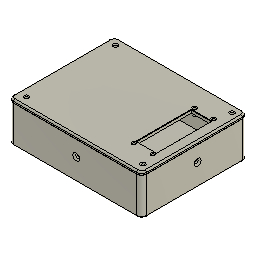
3d_case (Autodesk Fusion 360 design; units mm, degrees)
Autodesk Fusion 360 part; units mm, degrees
note: some values were not read from the file. Chosen so that the rebuilt part matches the saved one: which bodies a step acts on.
sketch "Sketch1" plane through (0, 0, 0) normal (0, 0, 1) x (1, 0, 0)
  line L0 (25.4, 25.4) -> (171.785, 25.4)
  line L1 (171.785, 25.4) -> (171.785, 136.054)
  line L2 (171.785, 136.054) -> (25.4, 136.054)
  line L3 (25.4, 136.054) -> (25.4, 25.4)
  line L4 (17.9, 15.4) -> (179.285, 15.4)
  line L5 (181.785, 17.9) -> (181.785, 143.554)
  line L6 (179.285, 146.054) -> (17.9, 146.054)
  line L7 (15.4, 143.554) -> (15.4, 17.9)
  arc A0 (17.9, 146.054) -> (15.4, 143.554) centre (17.9, 143.554) ccw
  arc A1 (15.4, 17.9) -> (17.9, 15.4) centre (17.9, 17.9) ccw
  arc A2 (179.285, 15.4) -> (181.785, 17.9) centre (179.285, 17.9) ccw
  arc A3 (181.785, 143.554) -> (179.285, 146.054) centre (179.285, 143.554) ccw
  line L8 (11.4, 143.554) -> (11.4, 17.9)
  arc A4 (11.4, 17.9) -> (17.9, 11.4) centre (17.9, 17.9) ccw
  line L9 (17.9, 11.4) -> (179.285, 11.4)
  arc A5 (179.285, 11.4) -> (185.785, 17.9) centre (179.285, 17.9) ccw
  line L10 (185.785, 17.9) -> (185.785, 143.554)
  arc A6 (185.785, 143.554) -> (179.285, 150.054) centre (179.285, 143.554) ccw
  line L11 (179.285, 150.054) -> (17.9, 150.054)
  arc A7 (17.9, 150.054) -> (11.4, 143.554) centre (17.9, 143.554) ccw
  dimension "d2" = 2.5
  dimension "d3" = 4
  constraint parallel L0 L4
  constraint parallel L1 L5
  constraint parallel L2 L6
  constraint parallel L3 L7
  constraint tangent L6 A0
  constraint tangent L7 A0
  constraint tangent L4 A1
  constraint tangent L7 A1
  constraint equal A0 A1
  constraint tangent L4 A2
  constraint tangent L5 A2
  constraint equal A0 A2
  constraint tangent L5 A3
  constraint tangent L6 A3
  constraint equal A0 A3
  measures "d2" radius of A0
extrude "Extrude1" add sketch "Sketch1" along normal blind 5 and the other way blind 40 contours L8 A4 L9 A5 L10 A6 L11 A7 makes body 1
extrude "Extrude2" add sketch "Sketch1" against normal blind 4 from surface at -40 contours L0 L1 L2 L3 | L4 L5 L6 L7 A0 A1 A2 A3 | L8 A4 L9 A5 L10 A6 L11 A7 bodies 1
extrude "Extrude3" add sketch "Sketch1" along normal blind 4 from surface at 5 separate body contours L0 L1 L2 L3 | L4 L5 L6 L7 A0 A1 A2 A3 | L8 A4 L9 A5 L10 A6 L11 A7 makes body 2
fillet "Fillet1" radius 2 16 edges at (98.5925, 150.054, -44) (183.8812, 148.1502, -44) (185.785, 80.727, -44) (183.8812, 13.3038, -44) (98.5925, 11.4, -44) (13.3038, 13.3038, -44) (11.4, 80.727, -44) (13.3038, 148.1502, -44) (11.4, 80.727, 9) (13.3038, 13.3038, 9) (98.5925, 11.4, 9) (183.8812, 13.3038, 9) (185.785, 80.727, 9) (183.8812, 148.1502, 9) (98.5925, 150.054, 9) (13.3038, 148.1502, 9) on bodies 1 2
fillet "Fillet2" radius 0.25 8 edges at (185.785, 80.727, 5) (183.8812, 148.1502, 5) (98.5925, 150.054, 5) (13.3038, 148.1502, 5) (11.4, 80.727, 5) (13.3038, 13.3038, 5) (98.5925, 11.4, 5) (183.8812, 13.3038, 5) on bodies 2
sketch "Sketch2" plane through (0, 0, 5) normal (0, 0, 1) x (-1, 0, 0)
  arc A0 (-181.785, -143.554) -> (-179.285, -146.054) centre (-179.285, -143.554) ccw
  line L0 (-181.785, -143.554) -> (-181.785, -17.9)
  arc A1 (-179.285, -15.4) -> (-181.785, -17.9) centre (-179.285, -17.9) ccw
  line L1 (-179.285, -15.4) -> (-17.9, -15.4)
  arc A2 (-15.4, -17.9) -> (-17.9, -15.4) centre (-17.9, -17.9) ccw
  line L2 (-15.4, -17.9) -> (-15.4, -143.554)
  arc A3 (-17.9, -146.054) -> (-15.4, -143.554) centre (-17.9, -143.554) ccw
  line L3 (-17.9, -146.054) -> (-179.285, -146.054)
  arc A4 (-17.9, -150.054) -> (-11.4, -143.554) centre (-17.9, -143.554) ccw
  line L4 (-11.4, -143.554) -> (-11.4, -17.9)
  arc A5 (-11.4, -17.9) -> (-17.9, -11.4) centre (-17.9, -17.9) ccw
  line L5 (-17.9, -11.4) -> (-179.285, -11.4)
  arc A6 (-179.285, -11.4) -> (-185.785, -17.9) centre (-179.285, -17.9) ccw
  line L6 (-185.785, -17.9) -> (-185.785, -143.554)
  arc A7 (-185.785, -143.554) -> (-179.285, -150.054) centre (-179.285, -143.554) ccw
  line L7 (-179.285, -150.054) -> (-17.9, -150.054)
  arc A8 (-17.9, -148.054) -> (-13.4, -143.554) centre (-17.9, -143.554) ccw
  line L8 (-13.4, -17.9) -> (-13.4, -143.554)
  arc A9 (-13.4, -17.9) -> (-17.9, -13.4) centre (-17.9, -17.9) ccw
  line L9 (-179.285, -13.4) -> (-17.9, -13.4)
  arc A10 (-179.285, -13.4) -> (-183.785, -17.9) centre (-179.285, -17.9) ccw
  line L10 (-183.785, -143.554) -> (-183.785, -17.9)
  arc A11 (-183.785, -143.554) -> (-179.285, -148.054) centre (-179.285, -143.554) ccw
  line L11 (-17.9, -148.054) -> (-179.285, -148.054)
  dimension "d18" = -2
extrude "Extrude4" cut sketch "Sketch2" against normal blind 2 contours A8 L8 A9 L9 A10 L10 A11 L11 bodies 1
extrude "Extrude5" add sketch "Sketch2" against normal blind 2 contours A8 L8 A9 L9 A10 L10 A11 L11 bodies 2
fillet "Fillet3" radius 0.2 8 edges at (98.5925, 148.054, 3) (182.467, 146.736, 3) (183.785, 80.727, 3) (182.467, 14.718, 3) (98.5925, 13.4, 3) (14.718, 14.718, 3) (13.4, 80.727, 3) (14.718, 146.736, 3) on bodies 2
sketch "Sketch10" plane through (0, 0, 9) normal (0, 0, 1) x (-1, 0, 0)
  line L0 (-13.4, -143.554) -> (-13.4, -17.9)
  arc A0 (-13.4, -17.9) -> (-17.9, -13.4) centre (-17.9, -17.9) ccw
  line L1 (-17.9, -13.4) -> (-179.285, -13.4)
  arc A1 (-179.285, -13.4) -> (-183.785, -17.9) centre (-179.285, -17.9) ccw
  line L2 (-183.785, -17.9) -> (-183.785, -143.554)
  arc A2 (-183.785, -143.554) -> (-179.285, -148.054) centre (-179.285, -143.554) ccw
  line L3 (-179.285, -148.054) -> (-17.9, -148.054)
  arc A3 (-17.9, -148.054) -> (-13.4, -143.554) centre (-17.9, -143.554) ccw
  line L4 (-158.9282, -148.054) -> (-158.9282, -13.4) construction
  line L5 (-172.0282, -44.727) -> (-145.8282, -44.727)
  line L6 (-145.8282, -44.727) -> (-145.8282, -116.727)
  line L7 (-145.8282, -116.727) -> (-172.0282, -116.727)
  line L8 (-172.0282, -116.727) -> (-172.0282, -44.727)
  line L9 (-172.0282, -44.727) -> (-145.8282, -116.727) construction
  line L10 (-145.8282, -44.727) -> (-172.0282, -116.727) construction
  point P0 (-158.9282, -80.727)
  dimension "d87" = 26.2
  dimension "d88" = 72
  constraint coincident L3 L4.start
  constraint coincident L1 L4.end
  constraint perpendicular L1 L4
  constraint horizontal L5
  constraint perpendicular L5 L6
  constraint parallel L5 L7
  constraint parallel L6 L8
  constraint coincident L9 P0
  constraint coincident L10 P0
  constraint midpoint L4 P0
  measures "d87" distance of L6.end L7.end
  measures "d88" distance of L5.end L6.end
sketch "Sketch4" plane through (11.4, 0, 0) normal (-1, 0, 0) x (0, -1, 0)
  line L0 (-143.554, -42) -> (-17.9, -42)
  line L1 (-17.9, -42) -> (-17.9, 5)
  line L2 (-17.9, 5) -> (-143.554, 5)
  line L3 (-143.554, 5) -> (-143.554, -42)
  line L4 (-143.554, -18.5) -> (-17.9, -18.5) construction
  line L5 (-66.727, -27) -> (-94.727, -27)
  line L6 (-94.727, -27) -> (-94.727, -10)
  line L7 (-94.727, -10) -> (-66.727, -10)
  line L8 (-66.727, -10) -> (-66.727, -27)
  line L9 (-66.727, -27) -> (-94.727, -10) construction
  line L10 (-94.727, -27) -> (-66.727, -10) construction
  circle A0 centre (-80.5064, -7.1438) radius 1
  circle A1 centre (-81, -30) radius 1
  point P0 (-80.727, -18.5)
  dimension "d29" = 28
  dimension "d30" = 17
  dimension "d31" = 2
  dimension "d32" = 2
  constraint midpoint L3 L4.start
  constraint midpoint L1 L4.end
  constraint horizontal L5
  constraint perpendicular L5 L6
  constraint parallel L5 L7
  constraint parallel L6 L8
  constraint coincident L9 P0
  constraint coincident L10 P0
  constraint midpoint L4 P0
  measures "d29" distance of L6.end L7.end
  measures "d30" distance of L5.end L6.end
  measures "d31" diameter of A0
  measures "d32" diameter of A1
extrude "Extrude12" cut sketch "Sketch10" against normal blind 10 contours L5 L6 L7 L8 bodies 2
extrude "Extrude7" cut sketch "Sketch4" against normal blind 14 contours L5 L6 L7 L8 | A0 | A1 bodies 1
sketch "Sketch5" plane through (181.785, 0, 0) normal (-1, 0, 0) x (0, -1, 0)
  line L0 (-17.9, 3) -> (-143.554, 3)
  line L1 (-143.554, 3) -> (-143.554, -40)
  line L2 (-143.554, -40) -> (-17.9, -40)
  line L3 (-17.9, -40) -> (-17.9, 3)
  circle A0 centre (-118.7918, -5.4) radius 1
  circle A1 centre (-41.7918, -5.4) radius 1
  circle A2 centre (-118.7918, -31.4) radius 1
  circle A3 centre (-41.7918, -31.4) radius 1
  circle A4 centre (-118.7918, -5.4) radius 1.75
  circle A5 centre (-41.7918, -5.4) radius 1.75
  circle A6 centre (-118.7918, -31.4) radius 1.75
  circle A7 centre (-41.7918, -31.4) radius 1.75
  dimension "d35" = 2
  dimension "d38" = 77
  dimension "d39" = -26
  dimension "d40" = 3.5
  constraint concentric A0 A4
  measures "d35" diameter of A0
  measures "d40" diameter of A4
sketch "Sketch6" plane through (0, 0, 0) normal (0, 0, 1) x (-1, 0, 0)
  line L0 (-25.4, -25.4) -> (-171.785, -25.4)
  line L1 (-171.785, -25.4) -> (-171.785, -136.054)
  line L2 (-171.785, -136.054) -> (-25.4, -136.054)
  line L3 (-25.4, -136.054) -> (-25.4, -25.4)
  circle A0 centre (-32, -130) radius 1.25
  circle A1 centre (-32, -130) radius 2
  circle A2 centre (-165, -130) radius 1.25
  circle A3 centre (-165, -130) radius 2
  circle A4 centre (-32, -33) radius 1.25
  circle A5 centre (-32, -33) radius 2
  circle A6 centre (-165, -33) radius 1.25
  circle A7 centre (-165, -33) radius 2
  dimension "d43" = 2.5
  dimension "d46" = -133
  dimension "d47" = 97
  constraint concentric A0 A1
  measures "d43" diameter of A0
extrude "Extrude9" add sketch "Sketch6" against normal up to surface (39.59 mm away) from surface at -0.41 separate body contours A1 | A3 | A5 | A7 makes body 3 at (163.0025, 129.9003, -13.6067) makes body 4 at (164.1774, 31.177, -26.8033) makes body 5 at (33.3965, 31.5683, -26.8033) makes body 6 at (30.8325, 128.3761, -26.8033)
combine "Combine1" operation add target body 1 tool bodies 3 4 5 6
sketch "Sketch7" plane through (0, 0, -40) normal (0, 0, 1) x (-1, 0, 0)
  circle A0 centre (-32, -33) radius 2
  circle A1 centre (-165, -130) radius 2
  line L0 (-179.285, -146.054) -> (-17.9, -146.054)
  arc A2 (-17.9, -146.054) -> (-15.4, -143.554) centre (-17.9, -143.554) ccw
  line L1 (-15.4, -143.554) -> (-15.4, -17.9)
  arc A3 (-15.4, -17.9) -> (-17.9, -15.4) centre (-17.9, -17.9) ccw
  line L2 (-17.9, -15.4) -> (-179.285, -15.4)
  arc A4 (-179.285, -15.4) -> (-181.785, -17.9) centre (-179.285, -17.9) ccw
  line L3 (-181.785, -17.9) -> (-181.785, -143.554)
  arc A5 (-181.785, -143.554) -> (-179.285, -146.054) centre (-179.285, -143.554) ccw
  circle A6 centre (-165, -33) radius 2
  circle A7 centre (-32, -130) radius 2
  circle A8 centre (-23, -140) radius 1.25
  circle A9 centre (-23, -140) radius 2
  circle A10 centre (-176, -140) radius 2
  circle A11 centre (-176, -140) radius 1.25
  circle A12 centre (-23, -23) radius 2
  circle A13 centre (-23, -23) radius 1.25
  circle A14 centre (-176, -23) radius 2
  circle A15 centre (-176, -23) radius 1.25
  dimension "d53" = 2.5
  dimension "d54" = 4
  dimension "d57" = -153
  dimension "d58" = 117
  constraint concentric A8 A9
  measures "d53" diameter of A8
  measures "d54" diameter of A9
extrude "Extrude10" add sketch "Sketch7" along normal blind 45 separate body contours A9 | A10 | A12 | A14 makes body 7 at (174.8325, 21.3761, -10) makes body 8 at (21.0025, 23.0997, -10) makes body 9 at (174.0025, 139.9003, -25) makes body 10 at (21.0025, 139.9003, -25)
combine "Combine2" operation add target body 1 tool bodies 10 8 9 7
extrude "Extrude11" cut 4 faces at (176.9573, 24.4594, 5) (174.2574, 139.9006, 5) (24.1641, 141.3004, 5) (21.2621, 23.1615, 5) along direction (0, 0, 1) blind 14 on bodies 1 bodies 2 makes body 11 at (21.7562, 22.8755, 7.6667) makes body 12 at (176.1554, 138.7597, 7.6667) makes body 13 at (176.1554, 21.7597, 7.6667) makes body 14 at (64.9107, 93.2423, 9)
delete_body "RemoveBody1" bodies 2
delete_body "RemoveBody2" bodies 11
delete_body "RemoveBody3" bodies 12
delete_body "RemoveBody4" bodies 13
fillet "Fillet4" radius 1 4 edges at (24.8647, 139.2768, 9) (24.8647, 22.2768, 9) (177.8647, 139.2768, 9) (177.8647, 22.2768, 9) on bodies 14
fillet "Fillet6" radius 1 8 edges at (11.4, 80.727, -10) (11.4, 94.727, -18.5) (11.4, 80.727, -27) (11.4, 66.727, -18.5) (13.4, 66.727, -27) (13.4, 66.727, -10) (13.4, 94.727, -27) (13.4, 94.727, -10) on bodies 1 14
fillet "Fillet6" radius 0.5 8 edges at (172.0282, 80.727, 9) (158.9282, 116.727, 9) (172.0282, 116.727, 7) (145.8282, 116.727, 7) (145.8282, 80.727, 9) (145.8282, 44.727, 7) (158.9282, 44.727, 9) (172.0282, 44.727, 7) on bodies 1 14
copy_body "Body->Comp1" bodies 1 removing the originals makes body 15 in component "Component"
copy_body "Body->Comp2" bodies 14 removing the originals makes body 16 in component "Component'"
sketch "Sketch9" plane through (0, 15.4, 0) normal (0, 1, 0) x (-1, 0, 0)
  line L0 (-17.9, 3) -> (-179.285, 3)
  line L1 (-179.285, 3) -> (-179.285, -40)
  line L2 (-179.285, -40) -> (-17.9, -40)
  line L3 (-17.9, -40) -> (-17.9, 3)
  circle A0 centre (-136.7918, -31.4) radius 1.75
  circle A1 centre (-136.7918, -31.4) radius 1
  circle A2 centre (-136.7918, -5.4) radius 1
  circle A3 centre (-59.7918, -5.4) radius 1
  circle A4 centre (-136.7918, -5.4) radius 1.75
  circle A5 centre (-59.7918, -31.4) radius 1
  circle A6 centre (-59.7918, -5.4) radius 1.75
  circle A7 centre (-59.7918, -31.4) radius 1.75
  dimension "d79" = 77
  dimension "d80" = -26
  dimension "d81" = 2
  dimension "d82" = 3.5
  constraint concentric A2 A4
  measures "d81" diameter of A2
  measures "d82" diameter of A4
sketch "Sketch11" plane through (0, 0, 5) normal (0, 0, -1) x (1, 0, 0)
  circle A0 centre (23, -140) radius 2
  circle A1 centre (176, -23) radius 2
  circle A2 centre (176, -140) radius 2
  circle A3 centre (23, -23) radius 2
  line L0 (145.8282, -116.227) -> (145.8282, -45.227)
  arc A4 (146.3282, -44.727) -> (145.8282, -45.227) centre (146.3282, -45.227) ccw
  line L1 (146.3282, -44.727) -> (171.5282, -44.727)
  arc A5 (172.0282, -45.227) -> (171.5282, -44.727) centre (171.5282, -45.227) ccw
  line L2 (172.0282, -45.227) -> (172.0282, -116.227)
  arc A6 (171.5282, -116.727) -> (172.0282, -116.227) centre (171.5282, -116.227) ccw
  line L3 (171.5282, -116.727) -> (146.3282, -116.727)
  arc A7 (145.8282, -116.227) -> (146.3282, -116.727) centre (146.3282, -116.227) ccw
  line L4 (15.4, -17.9) -> (15.4, -143.554)
  arc A8 (15.4, -143.554) -> (17.9, -146.054) centre (17.9, -143.554) ccw
  line L5 (17.9, -146.054) -> (179.285, -146.054)
  arc A9 (179.285, -146.054) -> (181.785, -143.554) centre (179.285, -143.554) ccw
  line L6 (181.785, -143.554) -> (181.785, -17.9)
  arc A10 (181.785, -17.9) -> (179.285, -15.4) centre (179.285, -17.9) ccw
  line L7 (179.285, -15.4) -> (17.9, -15.4)
  arc A11 (17.9, -15.4) -> (15.4, -17.9) centre (17.9, -17.9) ccw
  circle A12 centre (171, -41) radius 1
  circle A13 centre (171, -41) radius 1.75
  circle A14 centre (146, -41) radius 1.75
  circle A15 centre (171, -121) radius 1.75
  circle A16 centre (146, -121) radius 1.75
  circle A17 centre (146, -41) radius 1
  circle A18 centre (171, -121) radius 1
  circle A19 centre (146, -121) radius 1
  dimension "d93" = 3.5
  dimension "d96" = -25
  dimension "d97" = -80
  constraint concentric A12 A13
  measures "d93" diameter of A13
extrude "Extrude1'" add sketch "Sketch11" along normal blind 5 contours A13 | A14 | A15 | A16 bodies 16 in component "Component'"
extrude "Extrude1''" add sketch "Sketch9" along normal blind 5 contours A0 | A4 | A6 | A7 bodies 15 in component "Component"
extrude "Extrude2'" cut sketch "Sketch11" against normal blind 4 contours A12 | A13 | A14 | A15 | A16 | A17 | A18 | A19 bodies 16 in component "Component'"
fillet "Fillet1'" radius 1 4 edges at (144.3684, 121.6328, 9) (169.3684, 121.6328, 9) (144.3684, 41.6328, 9) (169.3684, 41.6328, 9) on bodies 16 in component "Component'"
extrude "Extrude2''" cut sketch "Sketch6" against normal blind 200 contours A0 | A2 | A4 | A6 bodies 15 in component "Component"
extrude "Extrude3'" cut sketch "Sketch7" against normal blind 50 contours A8 | A11 | A13 | A15 bodies 15 in component "Component"
fillet "Fillet1''" radius 1.5 8 edges at (33.1654, 33.452, -44) (24.1654, 23.452, -44) (166.1654, 33.452, -44) (177.1654, 23.452, -44) (177.1654, 140.452, -44) (166.1654, 130.452, -44) (33.1654, 130.452, -44) (24.1654, 140.452, -44) on bodies 15 in component "Component"
sketch "Sketch13" plane through (185.785, 0, 0) normal (1, 0, 0) x (0, 1, 0)
  line L0 (17.9, -42) -> (143.554, -42)
  line L1 (143.554, -42) -> (143.554, 5)
  line L2 (143.554, 5) -> (17.9, 5)
  line L3 (17.9, 5) -> (17.9, -42)
  circle A0 centre (85, -15) radius 2.5
  dimension "d125" = 5
  measures "d125" diameter of A0
extrude "Extrude4'" cut sketch "Sketch13" against normal blind 40 contours A0 bodies 15 in component "Component"
sketch "Sketch14" plane through (0, 11.4, 0) normal (0, -1, 0) x (1, 0, 0)
  line L0 (17.9, -42) -> (179.285, -42)
  line L1 (179.285, -42) -> (179.285, 5)
  line L2 (179.285, 5) -> (17.9, 5)
  line L3 (17.9, 5) -> (17.9, -42)
  circle A0 centre (100, -15) radius 2.5
  dimension "d126" = 5
  measures "d126" diameter of A0
extrude "Extrude5'" cut sketch "Sketch14" against normal blind 10 contours A0 bodies 15 in component "Component"
fillet "Fillet2'" radius 2 2 edges at (97.6692, 11.4, -14.096) (185.785, 82.6692, -14.096) on bodies 15 in component "Component"
component "Component" placed x (1, 0, 0) y (0, 1, 0) z (0, 0, 1) at (0, 0, 0)
component "Component'" placed x (1, 0, 0) y (0, 1, 0) z (0, 0, 1) at (0, 0, 0)
